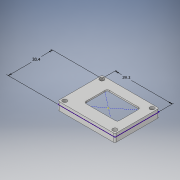
# Autodesk Inventor part: Enclosure_Lid
Saved by Autodesk Inventor 2019.4 (Build 234330000, 330)
## iProperties
Created: 2021-06-29
Part Number: Enclosure_Lid
Material: Generic
Document SubType Name: Modeling
Designer: keshav
Density: 1 g/cm^3
Appearance: Default
Author: keshav
Autodesk Inventor part; units mm, degrees
ref_plane "YZ Plane" through (0, 0, 0) normal (1, 0, 0) x (0, 1, 0)
ref_plane "XZ Plane" through (0, 0, 0) normal (0, 1, 0) x (-1, 0, 0)
ref_plane "XY Plane" through (0, 0, 0) normal (0, 0, 1) x (1, 0, 0)
sketch "Sketch1" plane through (0, 0, 0) normal (0, 1, 0) x (-1, 0, 0)
  line L0 (-19.65, 15.2) -> (19.65, 15.2)
  line L1 (19.65, 15.2) -> (19.65, -15.2)
  line L2 (19.65, -15.2) -> (-19.65, -15.2)
  line L3 (-19.65, -15.2) -> (-19.65, 15.2)
  line L4 (-19.65, 15.2) -> (19.65, -15.2) construction
  line L5 (19.65, 15.2) -> (-19.65, -15.2) construction
  point P0 (0, 0)
  dimension "d0" = 30.4
  dimension "d1" = 39.3
  constraints: 12 end point, 2 midpoint, 2 parallel, 1 horizontal, 1 perpendicular
  measures "d0" distance of L0.end L1.end
  measures "d1" distance of L1.end L2.end
extrude "Extrusion1" add sketch "Sketch1" along normal blind 2
sketch "Sketch2" plane through (0, 0, 0) normal (0, -1, 0) x (1, 0, 0)
  circle A0 centre (-17.225, -12.775) radius 2.425
  circle A1 centre (-17.225, -12.775) radius 1.475
  line L0 (-19.65, -15.2) -> (19.65, -15.2) projected
  line L1 (-19.65, 15.2) -> (-19.65, -15.2) projected
  circle A2 centre (-17.225, 12.775) radius 1.475
  circle A3 centre (-17.225, 12.775) radius 2.425
  circle A4 centre (17.225, 12.775) radius 1.475
  circle A5 centre (17.225, 12.775) radius 2.425
  circle A6 centre (17.225, -12.775) radius 1.475
  circle A7 centre (17.225, -12.775) radius 2.425
  line L2 (19.65, 15.2) -> (-19.65, 15.2) projected
  line L3 (19.65, -15.2) -> (19.65, 15.2) projected
  point P0 (0, 0)
  dimension "d4" = 0.95
  dimension "d5" = 2.95
  dimension "d6" = 2.95
  dimension "d7" = 0.95
  dimension "d8" = 2.95
  dimension "d9" = 0.95
  dimension "d10" = 2.95
  dimension "d11" = 0.95
  dimension "d12" = 39.3
  constraints: 8 centre point, 8 tangent, 4 coincident
  measures "d4" radial gap between concentric circles of A0 A1
  measures "d5" diameter of A1
  measures "d6" diameter of A2
  measures "d7" radial gap between concentric circles of A3 A2
  measures "d8" diameter of A4
  measures "d9" radial gap between concentric circles of A5 A4
  measures "d10" diameter of A6
  measures "d11" radial gap between concentric circles of A7 A6
  measures "d12" distance of L2.start L1.start
extrude "Extrusion3" add sketch "Sketch2" along normal blind 3.5 contours A0 | A3 | A7 | A5
sketch "Sketch3" plane through (0, 0, 0) normal (0, -1, 0) x (1, 0, 0)
  line L0 (-19.65, -15.2) -> (-17.225, -15.2) projected
  circle A0 centre (-17.225, 12.775) radius 2.425 projected
  line L1 (-19.65, -15.2) -> (-18.15, -15.2)
  line L2 (-18.15, -15.2) -> (-18.15, 15.0167)
  line L3 (-18.15, 15.0167) -> (-19.65, 15.0167)
  line L4 (-19.65, 15.0167) -> (-19.65, -15.2)
  point P0 (0, 0)
  dimension "d17" = 1.5
  constraints: 8 end point, 2 parallel, 1 horizontal, 1 perpendicular, 2 other
  measures "d17" distance of L3.end L2.end
extrude "Extrusion4" add sketch "Sketch3" along normal up to surface (3.5 mm away) contours L4 A0 L2 L0 | L4 L3 A0 | A0 L2 picked at (-18.7278, 13.0496)
sketch "Sketch4" plane through (0, 0, 0) normal (0, -1, 0) x (1, 0, 0)
  line L0 (19.65, -15.2) -> (-19.65, -15.2) projected
  line L1 (-19.65, -15.2) -> (-19.65, 15.2) projected
  line L2 (19.65, -15.2) -> (-19.65, -15.2)
  line L3 (-19.65, -15.2) -> (-19.65, -13.7)
  line L4 (-19.65, -13.7) -> (19.65, -13.7)
  line L5 (19.65, -13.7) -> (19.65, -15.2)
  point P0 (0, 0)
  dimension "d20" = 1.5
  constraints: 8 end point, 2 parallel, 1 horizontal, 1 perpendicular, 1 point on line
  measures "d20" distance of L2.end L3.end
extrude "Extrusion5" add sketch "Sketch4" along normal up to surface (3.5 mm away)
sketch "Sketch5" plane through (0, 0, 0) normal (0, -1, 0) x (1, 0, 0)
  line L0 (-19.65, 15.0167) -> (-19.65, -15.2) projected
  line L1 (19.65, 15.2) -> (-19.65, 15.2)
  line L2 (-19.65, 15.2) -> (-19.65, 14)
  line L3 (-19.65, 14) -> (19.65, 14)
  line L4 (19.65, 14) -> (19.65, 15.2)
  point P0 (0, 0)
  dimension "d23" = 1.2
  constraints: 8 end point, 2 parallel, 1 horizontal, 1 perpendicular, 1 point on line
  measures "d23" distance of L2.end L1.end
extrude "Extrusion6" add sketch "Sketch5" along normal up to surface (3.5 mm away)
sketch "Sketch6" plane through (0, 0, 0) normal (0, -1, 0) x (1, 0, 0)
  line L0 (-19.65, 15.2) -> (19.65, 15.2) projected
  line L1 (19.65, -15.2) -> (-19.65, -15.2) projected
  line L2 (19.65, 15.2) -> (18.45, 15.2)
  line L3 (18.45, 15.2) -> (18.45, -15.2)
  line L4 (18.45, -15.2) -> (19.65, -15.2)
  line L5 (19.65, -15.2) -> (19.65, 15.2)
  dimension "d27" = 1.2
  constraints: 8 end point, 2 parallel, 1 horizontal, 1 perpendicular, 1 point on line
  measures "d27" distance of L4.end L3.end
extrude "Extrusion7" add sketch "Sketch6" along normal up to surface (3.5 mm away)
sketch "Sketch7" plane through (0, -3.5, 0) normal (0, -1, 0) x (1, 0, 0)
  arc A0 (16.4034, 14) -> (18.45, 11.9534) centre (17.225, 12.775) ccw projected
  circle A1 centre (17.225, 12.775) radius 1.475
  arc A2 (18.45, -11.9534) -> (16.0761, -13.7) centre (17.225, -12.775) ccw projected
  circle A3 centre (17.225, -12.775) radius 1.475
  arc A4 (-16.0761, -13.7) -> (-18.15, -11.6261) centre (-17.225, -12.775) ccw projected
  circle A5 centre (-17.225, -12.775) radius 1.475
  arc A6 (-18.15, 11.6261) -> (-16.4034, 14) centre (-17.225, 12.775) ccw projected
  circle A7 centre (-17.225, 12.775) radius 1.475
  point P0 (0, 0)
  constraints: 4 centre point, 4 coincident
extrude "Extrusion8" cut sketch "Sketch7" against normal up to surface (5.5 mm away)
sketch "Sketch8" plane through (0, 2, 0) normal (0, 1, 0) x (1, 0, 0)
  line L0 (13.35, -7.2346) -> (-9.65, -7.2346)
  line L1 (-9.65, -7.2346) -> (-9.65, 8.7654)
  line L2 (-9.65, 8.7654) -> (13.35, 8.7654)
  line L3 (13.35, 8.7654) -> (13.35, -7.2346)
  line L4 (13.35, -7.2346) -> (-9.65, 8.7654) construction
  line L5 (-9.65, -7.2346) -> (13.35, 8.7654) construction
  line L6 (-19.65, 15.2) -> (-19.65, -15.2) projected
  point P0 (0, 0)
  point P1 (1.85, 0.7654)
  dimension "d34" = 23
  dimension "d35" = 10
  dimension "d40" = 16
  constraints: 12 end point, 2 midpoint, 2 parallel, 1 horizontal, 1 perpendicular
  measures "d34" distance of L1.end L2.end
  measures "d35" distance between parallel lines of L6 L1
  measures "d40" distance of L0.end L1.end
extrude "Extrusion9" cut sketch "Sketch8" against normal up to surface (2 mm away)
chamfer "Chamfer1" distance 1 angle 45 4 edges at (-9.65, 0, -0.7654) (1.85, 0, 7.2346) (13.35, 0, -0.7654) (1.85, 0, -8.7654)
fillet "Fillet2" radius 1 4 edges at (-19.65, -0.75, 15.2) (19.65, -0.75, 15.2) (19.65, -0.75, -15.2) (-19.65, -0.75, -15.2)
fillet "Fillet3" radius 1.5 4 edges at (13.35, 1.5, -8.7654) (-9.65, 1.5, -8.7654) (-9.65, 1.5, 7.2346) (13.35, 1.5, 7.2346)
body "Solid1"
